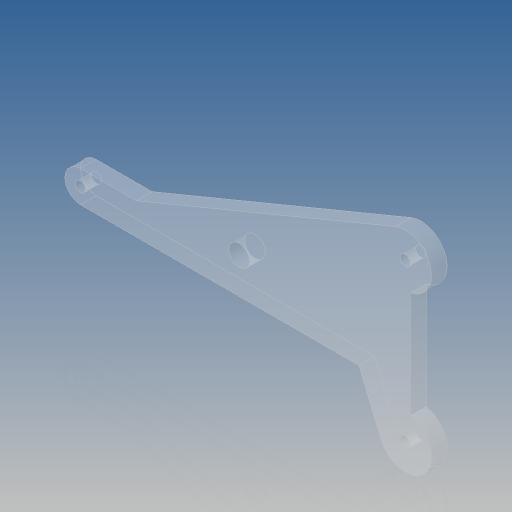
# Autodesk Inventor part: Protector
Saved by Autodesk Inventor 2017 (Build 210142000, 142)
## iProperties
Part Number: Protector
Material: Genérico
Document SubType Name: Modeling
Designer: Leo
Density: 1 g/cm^3
Appearance: Claro - Ligero
Author: Leo
Autodesk Inventor part; units mm, degrees
ref_plane "YZ Plane" through (0, 0, 0) normal (1, 0, 0) x (0, 1, 0)
ref_plane "XZ Plane" through (0, 0, 0) normal (0, 1, 0) x (-1, 0, 0)
ref_plane "XY Plane" through (0, 0, 0) normal (0, 0, 1) x (1, 0, 0)
sketch "Boceto1" plane through (0, 0, 0) normal (0, 0, 1) x (1, 0, 0)
  circle A0 centre (2.569, -31.6508) radius 2 projected
  circle A1 centre (126.296, -54.1016) radius 2 projected
  circle A2 centre (126.296, 5.8984) radius 2 projected
  line L0 (2.569, -25.6508) -> (23.8552, -25.6508)
  line L1 (23.8552, -25.6508) -> (122.4739, 15.1392)
  arc A3 (128.296, -3.8995) -> (122.4739, 15.1392) centre (126.296, 5.8984) ccw
  line L2 (128.296, -3.8995) -> (128.296, -44.3036)
  arc A4 (117.0553, -57.9237) -> (128.296, -44.3036) centre (126.296, -54.1016) ccw
  line L3 (117.0553, -57.9237) -> (108.6702, -37.6508)
  line L4 (108.6702, -37.6508) -> (2.569, -37.6508)
  arc A5 (2.569, -25.6508) -> (2.569, -37.6508) centre (2.569, -31.6508) ccw
  circle A6 centre (63.0505, -24.1016) radius 13.5492 construction
  circle A7 centre (63.0505, -24.1016) radius 4 projected
  point P0 (0, 0)
  dimension "d0" = 10
  dimension "d1" = 8
  dimension "d4" = 6
  constraints: 10 end point, 6 point on circle, 6 tangent, 4 centre point, 4 concentric, 2 perpendicular, 1 equal radius, 1 horizontal, 1 parallel
  measures "d0" radius of A3
  measures "d1" distance edge to line of A3 L2
  measures "d4" radius of A5
extrude "Extrusión1" add sketch "Boceto1" along normal blind 6
